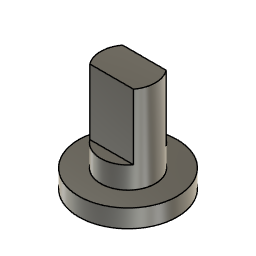
camisa+nueva (Autodesk Fusion 360 archive; units mm, degrees)
design "Eje motor"
Autodesk Fusion 360 part; units mm, degrees
sketch "Boceto1" plane through (0, 0, 0) normal (0, 0, 1) x (1, 0, 0)
  circle A0 centre (0, 0) radius 2.5
  line L0 (-2, 1.5) -> (2, 1.5)
  circle A1 centre (0, 0) radius 4.5
  line L1 (-2, -1.5) -> (2, -1.5)
  dimension "d1" = 5
  dimension "d2" = 1.5
  dimension "d3" = 9
  dimension "d10" = 3
  constraint coincident A0.centre A1.centre
  constraint coincident A0 L0.start
  constraint coincident A0 L0.end
  constraint horizontal L0
  constraint concentric A0 A1
  constraint coincident A0 L1.start
  constraint coincident A0 L1.end
  constraint horizontal L1
  measures "d1" diameter of A0
  measures "d2" distance of A0.centre L0
  measures "d3" diameter of A1
  measures "d10" distance of L0 L1
extrude "Extruir1" add sketch "Boceto1" along normal blind 8 contours A0 L0 L1 makes body 1
extrude "Extruir2" add sketch "Boceto1" along normal blind 2 contours A0 L0 | A0 L1 bodies 1
extrude "Extruir3" add sketch "Boceto1" against normal blind 1.65 separate body makes body 2
equation "d2 = d10 / 2"
